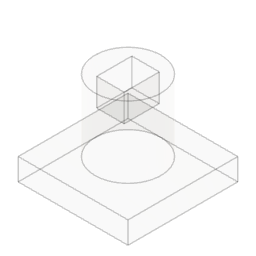
button2 (Autodesk Fusion 360 design; units mm, degrees)
Autodesk Fusion 360 part; units mm, degrees
sketch "Sketch1" plane through (0, 0, 0) normal (0, 0, 1) x (1, 0, 0)
  line L0 (0, 0) -> (10, 0)
  line L1 (10, 0) -> (10, 10)
  line L2 (10, 10) -> (0, 10)
  line L3 (0, 10) -> (0, 0)
  circle A0 centre (5, 5) radius 3
  dimension "d1" = 10
  dimension "d2" = 10
  dimension "d3" = 6
  constraint horizontal L0
  constraint vertical L1
  constraint horizontal L2
  constraint vertical L3
  constraint coincident L0.start L3.end
  measures "d1" distance of L0.start L0.end
  measures "d2" distance of L0.start L2.end
  measures "d3" diameter of A0
extrude "Extrude1" add sketch "Sketch1" along normal blind 2 contours L0 L1 L2 L3 | A0 makes body 1
extrude "Extrude2" add sketch "Sketch1" along normal blind 6 contours A0 bodies 1
sketch "Sketch2" plane through (0, 0, 6) normal (0, 0, 1) x (-1, 0, 0)
  circle A0 centre (-5, -5) radius 3
  line L0 (-5, -5) -> (-6.25, -5)
  line L1 (-6.25, -5) -> (-6.25, -3.4)
  line L2 (-6.25, -3.4) -> (-5, -3.4)
  line L3 (-5, -3.4) -> (-5, -5)
  line L4 (-5, -5) -> (-3.75, -5)
  line L5 (-3.75, -5) -> (-3.75, -6.6)
  line L6 (-3.75, -6.6) -> (-5, -6.6)
  line L7 (-5, -6.6) -> (-5, -5)
  line L8 (-3.75, -6.6) -> (-6.25, -6.6)
  line L9 (-6.25, -6.6) -> (-6.25, -3.4)
  line L10 (-6.25, -3.4) -> (-3.75, -3.4)
  line L11 (-3.75, -3.4) -> (-3.75, -6.6)
  dimension "d8" = 1.25
  dimension "d9" = 1.6
  dimension "d10" = 1.6
  constraint horizontal L0
  constraint vertical L1
  constraint horizontal L2
  constraint vertical L3
  constraint coincident A0.centre L0.start
  constraint horizontal L4
  constraint vertical L5
  constraint horizontal L6
  constraint vertical L7
  constraint horizontal L8
  constraint vertical L9
  constraint horizontal L10
  constraint vertical L11
  measures "d8" distance of A0.centre L0.end
  measures "d9" distance of A0.centre L2.end
  measures "d10" distance of A0.centre L6.end
extrude "Extrude3" add sketch "Sketch2" along normal blind 2.5 bodies 1
copy_body "Body->Comp1" bodies 1 removing the originals makes body 2 in component "Button"
sketch "Sketch1 (2)" plane through (0, 0, 0) normal (0, 0, 1) x (1, 0, 0) in component "Top"
  line L0 (0, 0) -> (20, 0)
  line L1 (20, 0) -> (20, 20)
  line L2 (20, 20) -> (0, 20)
  line L3 (0, 20) -> (0, 0)
  circle A0 centre (10, 10) radius 4.2
  line L4 (5.5, 14.5) -> (14.5, 14.5)
  line L5 (14.5, 14.5) -> (14.5, 5.5)
  line L6 (14.5, 5.5) -> (5.5, 5.5)
  line L7 (5.5, 5.5) -> (5.5, 14.5)
  line L8 (4.5, 15.5) -> (15.5, 15.5)
  line L9 (15.5, 15.5) -> (15.5, 4.5)
  line L10 (15.5, 4.5) -> (4.5, 4.5)
  line L11 (4.5, 4.5) -> (4.5, 15.5)
  dimension "d13" = 20
  dimension "d14" = 20
  dimension "d15" = 8.4
  dimension "d16" = 9
  dimension "d17" = 9
  dimension "d18" = 5.5
  dimension "d19" = 5.5
  dimension "d20" = 1
  dimension "d21" = 1
  dimension "d22" = 1
  dimension "d23" = 1
  constraint horizontal L0
  constraint vertical L1
  constraint horizontal L2
  constraint vertical L3
  constraint coincident L0.start L3.end
  constraint horizontal L4
  constraint vertical L5
  constraint horizontal L6
  constraint vertical L7
  constraint horizontal L8
  constraint vertical L9
  constraint horizontal L10
  constraint vertical L11
  measures "d13" distance of L0.start L0.end
  measures "d14" distance of L0.start L2.end
  measures "d15" diameter of A0
  measures "d16" distance of L4.start L4.end
  measures "d17" distance of L4.start L6.end
  measures "d18" distance of L2 L4
  measures "d19" distance of L3 L7
  measures "d20" distance of L4 L8
  measures "d21" distance of L7 L11
  measures "d22" distance of L5 L9
  measures "d23" distance of L6 L10
extrude "Extrude1'" add sketch "Sketch1 (2)" along normal blind 2 separate body makes body 3 at (1.5, 11.8333, 0) makes body 4 at (14.1948, 9.7906, 1.3333) in component "Top"
extrude "Extrude2'" add sketch "Sketch1 (2)" along normal blind 15.5 contours L8 L9 L10 L11 bodies 3 4 in component "Top"
extrude "Extrude3'" add 1 faces at (6.6008, 6.4532, 2) along direction (0, 0, 1) blind 4 on bodies 3 bodies 3 in component "Top"
extrude "Extrude4" add 1 faces at (6.6008, 6.4532, 6) along direction (0, 0, 1) blind 0.5 on bodies 3 bodies 3 in component "Top"
sketch "Sketch2 (2)" plane through (0, 0, 0) normal (0, 0, 1) x (1, 0, 0) in component "Top"
  line L0 (-25, 15) -> (-11.6, 15)
  line L1 (-11.6, 15) -> (-11.6, 1.6)
  line L2 (-11.6, 1.6) -> (-25, 1.6)
  line L3 (-25, 1.6) -> (-25, 15)
  line L4 (-24, 14) -> (-12.6, 14)
  line L5 (-12.6, 14) -> (-12.6, 2.6)
  line L6 (-12.6, 2.6) -> (-24, 2.6)
  line L7 (-24, 2.6) -> (-24, 14)
  line L8 (-22.8, 3.8) -> (-13.8, 3.8)
  line L9 (-13.8, 3.8) -> (-13.8, 12.8)
  line L10 (-13.8, 12.8) -> (-22.8, 12.8)
  line L11 (-22.8, 12.8) -> (-22.8, 3.8)
  line L12 (-13.8, 12.8) -> (-16.8, 12.8)
  line L13 (-16.8, 12.8) -> (-16.8, 7.8)
  line L14 (-16.8, 7.8) -> (-13.8, 7.8)
  line L15 (-13.8, 7.8) -> (-13.8, 12.8)
  dimension "d32" = 13.4
  dimension "d33" = 13.4
  dimension "d34" = 11.4
  dimension "d35" = 11.4
  dimension "d36" = 9
  dimension "d37" = 9
  dimension "d38" = 1.2
  dimension "d39" = 1.2
  dimension "d40" = 3
  dimension "d41" = 5
  constraint horizontal L0
  constraint vertical L1
  constraint horizontal L2
  constraint vertical L3
  constraint horizontal L4
  constraint vertical L5
  constraint horizontal L6
  constraint vertical L7
  constraint horizontal L8
  constraint vertical L9
  constraint horizontal L10
  constraint vertical L11
  constraint horizontal L12
  constraint vertical L13
  constraint horizontal L14
  constraint vertical L15
  measures "d32" distance of L0.start L0.end
  measures "d33" distance of L0.start L2.end
  measures "d34" distance of L4.start L4.end
  measures "d35" distance of L4.start L6.end
  measures "d36" distance of L8.start L8.end
  measures "d37" distance of L8.start L10.end
  measures "d38" distance of L6.end L8
  measures "d39" distance of L7 L11
  measures "d40" distance of L9.end L12.end
  measures "d41" distance of L9.end L14.end
sketch "Sketch3" plane through (4.5, 0, 0) normal (-1, 0, 0) x (0, -1, 0) in component "Top"
  line L0 (-15.5, 2) -> (-4.5, 2)
  line L1 (-4.5, 2) -> (-4.5, 15.5)
  line L2 (-4.5, 15.5) -> (-15.5, 15.5)
  line L3 (-15.5, 15.5) -> (-15.5, 2)
  line L4 (-15.5, 15.5) -> (-4.5, 15.5)
  line L5 (-4.5, 15.5) -> (-4.5, 19.5)
  line L6 (-4.5, 19.5) -> (-15.5, 19.5)
  line L7 (-15.5, 19.5) -> (-15.5, 15.5)
  circle A0 centre (-10, 17) radius 1.5
  dimension "d46" = 4
  dimension "d47" = 3
  constraint horizontal L4
  constraint vertical L5
  constraint horizontal L6
  constraint vertical L7
  constraint coincident L2.end L3.start
  measures "d46" distance of L2.end L6.end
  measures "d47" diameter of A0
extrude "Extrude7" add sketch "Sketch3" against normal blind 1 contours L2 L4 L5 L6 L7 bodies 3 in component "Top"
sketch "Sketch4" plane through (5.5, 0, 0) normal (1, 0, 0) x (0, 1, 0) in component "Top"
  line L0 (5.5, 15.5) -> (5.5, 6.5)
  line L1 (5.5, 6.5) -> (14.5, 6.5)
  line L2 (14.5, 6.5) -> (14.5, 15.5)
  line L3 (14.5, 15.5) -> (15.5, 15.5)
  line L4 (15.5, 15.5) -> (15.5, 19.5)
  line L5 (15.5, 19.5) -> (4.5, 19.5)
  line L6 (4.5, 19.5) -> (4.5, 15.5)
  line L7 (4.5, 15.5) -> (5.5, 15.5)
  circle A0 centre (10, 17) radius 1.5
  line L8 (4.5, 19.5) -> (5.5, 19.5)
  line L9 (5.5, 19.5) -> (5.5, 15.5)
  line L10 (5.5, 15.5) -> (4.5, 15.5)
  line L11 (4.5, 15.5) -> (4.5, 19.5)
  line L12 (15.5, 19.5) -> (14.5, 19.5)
  line L13 (14.5, 19.5) -> (14.5, 15.5)
  line L14 (14.5, 15.5) -> (15.5, 15.5)
  line L15 (15.5, 15.5) -> (15.5, 19.5)
  dimension "d50" = 1
  dimension "d51" = 4
  constraint horizontal L8
  constraint vertical L9
  constraint horizontal L10
  constraint vertical L11
  constraint coincident L0.start L7.end
  constraint coincident L5.end L6.start
  constraint horizontal L12
  constraint vertical L13
  constraint horizontal L14
  constraint vertical L15
  constraint coincident L4.end L5.start
  measures "d50" distance of L4.end L12.end
  measures "d51" distance of L4.end L3.end
extrude "Extrude8" add sketch "Sketch4" along normal blind 9 contours L5 L6 L7 L8 L9 L10 L11 | L3 L4 L5 L12 L13 L14 L15 bodies 3 in component "Top"
sketch "Sketch5" plane through (14.5, 0, 0) normal (1, 0, 0) x (0, 1, 0) in component "Top"
  line L0 (4.5, 15.5) -> (5.5, 15.5)
  line L1 (5.5, 15.5) -> (5.5, 19.5)
  line L2 (5.5, 19.5) -> (4.5, 19.5)
  line L3 (4.5, 19.5) -> (4.5, 15.5)
  line L4 (4.5, 19.5) -> (15.5, 19.5)
  line L5 (15.5, 19.5) -> (15.5, 15.5)
  line L6 (15.5, 15.5) -> (4.5, 15.5)
  line L7 (4.5, 15.5) -> (4.5, 19.5)
  circle A0 centre (10, 17) radius 1.5
  dimension "d54" = 3
  constraint horizontal L4
  constraint vertical L5
  constraint horizontal L6
  constraint vertical L7
  constraint coincident L2.end L3.start
  measures "d54" diameter of A0
extrude "Extrude9" add sketch "Sketch5" along normal blind 1 bodies 3 in component "Top"
component "Button" placed x (1, 0, 0) y (0, 1, 0) z (0, 0, 1) at (0, 0, 0)
component "Top" placed x (1, 0, 0) y (0, 1, 0) z (0, 0, 1) at (0, 0, 0)
